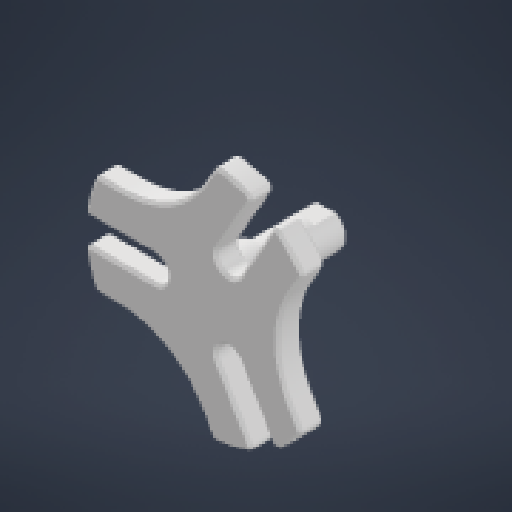
# Autodesk Inventor part: geniva2
Saved by Autodesk Inventor 2026.3 (Build 303398000, 398)
## iProperties
Created: 2026-04-30
Part Number: geniva2
Material: Generic
Document SubType Name: Modeling
Designer: frede
Density: 1 g/cm^3
Appearance: Default
Author: frede
Autodesk Inventor part; units mm, degrees
ref_plane "YZ Plane" through (0, 0, 0) normal (1, 0, 0) x (0, 1, 0)
ref_plane "XZ Plane" through (0, 0, 0) normal (0, 1, 0) x (-1, 0, 0)
ref_plane "XY Plane" through (0, 0, 0) normal (0, 0, 1) x (1, 0, 0)
sketch "Sketch1" plane through (0, 0, 0) normal (0, 0, 1) x (1, 0, 0)
  circle A0 centre (0, 0) radius 10.36
  arc A1 (-10.36, -2.6) -> (-10.36, 2.6) centre (-10.36, 0) ccw
  line L0 (-10.36, 2.6) -> (-24.8644, 2.6)
  line L1 (-10.36, -2.6) -> (-24.8644, -2.6)
  arc A2 (7.4317, -7.672) -> (2.9283, -10.272) centre (5.18, -8.972) ccw
  line L2 (2.9283, -10.272) -> (10.1806, -22.8332)
  line L3 (7.4317, -7.672) -> (14.6839, -20.2332)
  arc A3 (2.9283, 10.272) -> (7.4317, 7.672) centre (5.18, 8.972) ccw
  line L4 (7.4317, 7.672) -> (14.6839, 20.2332)
  line L5 (2.9283, 10.272) -> (10.1806, 22.8332)
  line L6 (-10.36, 2.6) -> (2.783, 9.9792)
  line L7 (0, 0) -> (-17.3112, 30.8327)
  arc A4 (-17.3112, 10.8327) -> (-0.2357, 20.4198) centre (-17.3112, 30.8327) ccw
  line L8 (-17.3112, 10.8327) -> (-22.5312, 10.8327)
  line L9 (-0.2357, 20.4198) -> (2.4821, 24.8765)
  line L10 (-17.5662, -10.414) -> (-22.7847, -10.2887)
  arc A5 (-0.7258, -20.4082) -> (-17.5662, -10.414) centre (-18.0463, -30.4082) ccw
  line L11 (-0.7258, -20.4082) -> (1.8842, -24.9289)
  line L12 (17.8019, -10.0058) -> (20.3026, -14.5878)
  arc A6 (18.0369, 9.5756) -> (17.8019, -10.0058) centre (35.3575, -0.4244) ccw
  line L13 (18.0369, 9.5756) -> (20.6469, 14.0962)
  arc A7 (20.6469, 14.0962) -> (14.6839, 20.2332) centre (0, 0) ccw
  arc A8 (10.1806, 22.8332) -> (2.4821, 24.8765) centre (0, 0) ccw
  arc A9 (-22.5312, 10.8327) -> (-24.8644, 2.6) centre (0, 0) ccw
  arc A10 (-24.8644, -2.6) -> (-22.7847, -10.2887) centre (0, 0) ccw
  arc A11 (1.8842, -24.9289) -> (10.1806, -22.8332) centre (0, 0) ccw
  arc A12 (14.6839, -20.2332) -> (20.3026, -14.5878) centre (0, 0) ccw
  point P0 (-24.0472, 10.8327)
  point P1 (3.2714, 26.1708)
  dimension "d1" = 20.72
  dimension "d2" = 5.2
  dimension "d5" = 360
  dimension "d7" = 35.36
  dimension "d8" = 40
  dimension "d11" = 360
  constraints: 28 end point, 27 point on circle, 13 centre point, 3 coincident, 3 horizontal, 3 tangent, 2 symmetric about line, 1 perpendicular, 50 other
  measures "d1" diameter of A0
  measures "d2" diameter of A1
  measures "d7" distance of L7.start L7.end
  measures "d8" diameter of A4
extrude "Extrusion1" add sketch "Sketch1" along normal blind 5 contours A0 A2 A1 L6 A3 | A0 A3 L4 A7 L13 A6 L12 A12 L3 A2 | L6 L7 A0 | A0 L7 A4 L9 A8 L5 A3 | A2 L2 A11 L11 A5 L10 A10 L1 A1 A0 | L7 L6 A0 | A0 L6 L0 A9 L8 A4 L7 | A0 A1 L6
sketch "Sketch2" plane through (0, 0, 0) normal (0, 0, -1) x (-1, 0, 0)
  circle A0 centre (0, 0) radius 5
  dimension "d15" = 10
  constraints: 1 centre point, 1 coincident
  measures "d15" diameter of A0
extrude "Extrusion2" add sketch "Sketch2" along normal blind 6.1
sketch "Sketch3" plane through (0, 0, -6.1) normal (0, 0, -1) x (-1, 0, 0)
  circle A0 centre (0, 0) radius 5 projected
  circle A1 centre (0, 0) radius 4
  point P0 (-3.5, 1.9365)
  point P1 (-3.5, -1.9365)
  dimension "d18" = 8
  constraints: 2 point on circle, 1 centre point, 1 coincident
  measures "d18" diameter of A1
extrude "Extrusion3" add sketch "Sketch3" along normal blind 15 contours A1
fillet "Fillet1" radius 0.5 1 edges at (5, 0, 0)
fillet "Fillet2" radius 1 12 edges at (-24.8644, 2.6, 2.5) (-24.8644, -2.6, 2.5) (10.1806, -22.8332, 2.5) (14.6839, -20.2332, 2.5) (14.6839, 20.2332, 2.5) (10.1806, 22.8332, 2.5) (-22.5312, 10.8327, 2.5) (-22.7847, -10.2887, 2.5) (1.8842, -24.9289, 2.5) (20.3026, -14.5878, 2.5) (20.6469, 14.0962, 2.5) (2.4821, 24.8765, 2.5)
chamfer "Chamfer2" distance 0.6 angle 45 72 edges at (3.88, -6.7204, 5) (10.7738, -13.4607, 5) (14.7965, -19.7321, 5) (17.898, -17.4546, 5) (20.1165, -14.5817, 5) (18.8995, -12.0169, 5) (15.3589, -0.1844, 5) (19.1825, 11.5597, 5) (20.4607, 14.0946, 5) (18.1062, 17.2385, 5) (14.7965, 19.7321, 5) (10.7738, 13.4607, 5) (3.88, 6.7204, 5) (6.2704, 16.0607, 5) (9.6903, 22.6802, 5) (6.1671, 24.2274, 5) (2.5699, 24.7122, 5) (0.9572, 22.3759, 5) (-7.5198, 13.3934, 5) (-19.6022, 10.8327, 5) (-22.4366, 10.6722, 5) (-23.9821, 7.0612, 5) (-24.4868, 2.9481, 5) (-17.0442, 2.6, 5) (-7.76, 0, 5) (-17.0442, -2.6, 5) (-24.4868, -2.9481, 5) (-24.0651, -6.7728, 5) (-22.6863, -10.1306, 5) (-19.8566, -10.359, 5) (-7.8391, -13.209, 5) (0.4198, -22.3924, 5) (1.9759, -24.7668, 5) (5.8759, -24.2997, 5) (9.6903, -22.6802, 5) (6.2704, -16.0607, 5) (3.88, -6.7204, 0) (10.7738, -13.4607, 0) (14.7965, -19.7321, 0) (17.898, -17.4546, 0) (20.1165, -14.5817, 0) (18.8995, -12.0169, 0) (15.3589, -0.1844, 0) (19.1825, 11.5597, 0) (20.4607, 14.0946, 0) (18.1062, 17.2385, 0) (14.7965, 19.7321, 0) (10.7738, 13.4607, 0) (3.88, 6.7204, 0) (6.2704, 16.0607, 0) (9.6903, 22.6802, 0) (6.1671, 24.2274, 0) (2.5699, 24.7122, 0) (0.9572, 22.3759, 0) (-7.5198, 13.3934, 0) (-19.6022, 10.8327, 0) (-22.4366, 10.6722, 0) (-23.9821, 7.0612, 0) (-24.4868, 2.9481, 0) (-17.0442, 2.6, 0) (-7.76, 0, 0) (-17.0442, -2.6, 0) (-24.4868, -2.9481, 0) (-24.0651, -6.7728, 0) (-22.6863, -10.1306, 0) (-19.8566, -10.359, 0) (-7.8391, -13.209, 0) (0.4198, -22.3924, 0) (1.9759, -24.7668, 0) (5.8759, -24.2997, 0) (9.6903, -22.6802, 0) (6.2704, -16.0607, 0)
fillet "Fillet4" radius 0.5 1 edges at (4, 0, -6.1)
sketch "Sketch7" plane through (0, 0, -21.1) normal (0, 0, -1) x (-1, 0, 0)
  arc A0 (1.9365, 3.5) -> (-1.9365, 3.5) centre (0, 0) ccw
  line L0 (-1.9365, 3.5) -> (1.9365, 3.5)
  constraints: 2 end point, 2 point on circle, 1 centre point, 1 coincident, 1 horizontal
extrude "Extrusion6" cut sketch "Sketch7" against normal blind 5
chamfer "Chamfer6" distance 0.5 angle 45 3 edges at (0, 3.5, -21.1) (2.0315, -3.4457, -21.1) (-3.4457, 2.0315, -21.1)
chamfer "Chamfer7" distance 0.25 angle 45 1 edges at (5, 0, -6.1)
body "Solid1"
